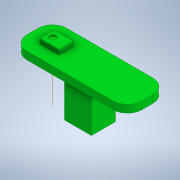
# Autodesk Inventor part: Mikrofonboard
Saved by Autodesk Inventor 2020.2 (Build 242310000, 310)
## iProperties
Created: 2020-02-12
Part Number: Mikrofonboard
Material: Generisch
Document SubType Name: Modeling
Designer: Max
Density: 1 g/cm^3
Appearance: Vorgabe
Author: Max
Autodesk Inventor part; units mm, degrees
ref_plane "YZ Plane" through (0, 0, 0) normal (1, 0, 0) x (0, 1, 0)
ref_plane "XZ Plane" through (0, 0, 0) normal (0, 1, 0) x (-1, 0, 0)
ref_plane "XY Plane" through (0, 0, 0) normal (0, 0, 1) x (1, 0, 0)
sketch "Skizze1" plane through (0, 0, 0) normal (0, 1, 0) x (-1, 0, 0)
  line L0 (9, -4.15) -> (-9, -4.15)
  line L1 (-12, -1.15) -> (-12, 1.15)
  line L2 (-9, 4.15) -> (9, 4.15)
  line L3 (12, 1.15) -> (12, -1.15)
  line L4 (0, -12.6778) -> (0, 8.6418)
  line L5 (13.6706, 0) -> (-20.1804, 0)
  arc A0 (9, -4.15) -> (12, -1.15) centre (9, -1.15) ccw
  arc A1 (12, 1.15) -> (9, 4.15) centre (9, 1.15) ccw
  arc A2 (-9, 4.15) -> (-12, 1.15) centre (-9, 1.15) ccw
  arc A3 (-12, -1.15) -> (-9, -4.15) centre (-9, -1.15) ccw
  point P0 (0, 0)
  point P1 (12, -4.15)
  point P2 (-12, -4.15)
  dimension "d0" = 8.3
  dimension "d1" = 24
  dimension "d2" = 3
  constraints: 12 end point, 8 point on circle, 8 tangent, 6 point on line, 4 centre point, 3 equal radius, 2 horizontal, 2 parallel, 1 perpendicular, 1 vertical, 2 other
  measures "d0" distance between parallel lines of L2 L0
  measures "d1" distance of point (12, -4.15) point (-12, -4.15)
  measures "d2" radius of A0
extrude "Extrusion1" add sketch "Skizze1" along normal blind 1.6
sketch "Skizze2" plane through (0, 0, 0) normal (0, -1, 0) x (1, 0, 0)
  line L0 (-2.8, 2.5) -> (2.8, 2.5)
  line L1 (2.8, 2.5) -> (2.8, -2.5)
  line L2 (2.8, -2.5) -> (-2.8, -2.5)
  line L3 (-2.8, -2.5) -> (-2.8, 2.5)
  line L4 (-9.3724, 0) -> (8.2101, 0)
  line L5 (0, 7.7773) -> (0, -6.9118)
  point P0 (0, 0)
  dimension "d5" = 5.6
  dimension "d6" = 5
  constraints: 12 end point, 2 horizontal, 2 parallel, 2 point on line, 1 perpendicular, 1 vertical, 2 other
  measures "d5" distance of L1.end L2.end
  measures "d6" distance of L0.end L1.end
extrude "Extrusion2" add sketch "Skizze2" along normal blind 8.6
sketch "Skizze3" plane through (0, 1.6, 0) normal (0, 1, 0) x (1, 0, 0)
  line L0 (-9, 1.5) -> (-5, 1.5)
  line L1 (-5, 1.5) -> (-5, -1.5)
  line L2 (-5, -1.5) -> (-9, -1.5)
  line L3 (-9, -1.5) -> (-9, 1.5)
  line L4 (-9.8398, 0) -> (1.393, 0)
  line L5 (-12, 1.15) -> (-12, -1.15) projected
  point P0 (0, 0)
  dimension "d9" = 3
  dimension "d10" = 4
  dimension "d11" = 3
  constraints: 10 end point, 2 horizontal, 2 parallel, 1 perpendicular, 1 point on line, 1 other
  measures "d9" distance of L0.end L1.end
  measures "d10" distance of L1.end L2.end
  measures "d11" distance between parallel lines of L5 L3
extrude "Extrusion3" add sketch "Skizze3" along normal blind 1
sketch "Skizze4" plane through (0, 2.6, 0) normal (0, 1, 0) x (1, 0, 0)
  circle A0 centre (-7.78, 0) radius 0.65
  line L0 (-5, 1.5) -> (-9, 1.5) projected
  line L1 (-5, -1.5) -> (-5, 1.5) projected
  point P0 (0, 0)
  dimension "d14" = 1.3
  dimension "d15" = 1.5
  dimension "d16" = 2.78
  constraints: 1 centre point
  measures "d14" diameter of A0
  measures "d15" distance from line of L0 A0.centre
  measures "d16" distance from line of A0.centre L1
extrude "Extrusion4" cut sketch "Skizze4" against normal blind 0.2
